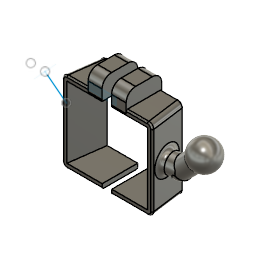
Titan_Grab_Bar_Monitor_Mount 2 v1.1 (Autodesk Fusion 360 design; units mm, degrees)
part number: 2026-08-07-00-05-41-022
Autodesk Fusion 360 part; units mm, degrees
sketch "Sketch1" plane through (0, 0, 0) normal (0, 0, 1) x (1, 0, 0)
  line L0 (19.05, -19.05) -> (-19.05, -19.05)
  line L1 (-19.05, -19.05) -> (-19.05, 19.05)
  line L2 (-19.05, 19.05) -> (19.05, 19.05)
  line L3 (19.05, 19.05) -> (19.05, -19.05)
  line L4 (19.05, -19.05) -> (-19.05, 19.05) construction
  line L5 (-19.05, -19.05) -> (19.05, 19.05) construction
  dimension "d8" = 38.1
  dimension "d9" = 38.1
  constraint horizontal L0
  constraint perpendicular L0 L1
  constraint parallel L0 L2
  constraint parallel L1 L3
  constraint coincident L4 origin
  constraint coincident L5 origin
  measures "d8" distance of L1.end L2.end
  measures "d9" distance of L0.end L1.end
ref_plane "WorkPlane1" through (0, 0, 19.05) normal (0, 0, 1) x (1, 0, 0)
sketch "Sketch2" plane through (0, 0, 19.05) normal (0, 0, 1) x (1, 0, 0)
  line L0 (16.51, 19.05) -> (-16.51, 19.05)
  line L1 (-16.51, 19.05) -> (-16.51, -19.05)
  line L2 (-16.51, -19.05) -> (16.51, -19.05)
  line L3 (16.51, -19.05) -> (16.51, 19.05)
  line L4 (16.51, 19.05) -> (-16.51, -19.05) construction
  line L5 (-16.51, 19.05) -> (16.51, -19.05) construction
  dimension "d12" = 33.02
  dimension "d13" = 38.1
  constraint horizontal L0
  constraint perpendicular L0 L1
  constraint parallel L0 L2
  constraint parallel L1 L3
  constraint coincident L4 origin
  constraint coincident L5 origin
  measures "d12" distance of L1.end L2.end
  measures "d13" distance of L0.end L1.end
loft "Loft1" add profiles "Sketch1", "Sketch2" section 1 section 2 makes body 1
shell "Shell3" thickness 2.54 outward yes removed faces 2 at (5.5033, -6.35, 19.05) at (-6.35, 6.35, 0) on bodies 1
fillet "Fillet1" radius 2.54 4 edges at (-20.3425, 21.59, 9.525) (20.3425, 21.59, 9.525) (20.3425, -21.59, 9.525) (-20.3425, -21.59, 9.525) on bodies 1
fillet "Fillet2" radius 0.762 24 edges at (19.0725, 0, 19.05) (18.3219, -20.8461, 19.05) (0, -21.59, 19.05) (-18.3219, -20.8461, 19.05) (-19.0725, 0, 19.05) (-18.3219, 20.8461, 19.05) (0, 21.59, 19.05) (18.3219, 20.8461, 19.05) (20.8619, 20.8461, 0) (21.6125, 0, 0) (20.8619, -20.8461, 0) (0, -21.59, 0) (-20.8619, -20.8461, 0) (-21.6125, 0, 0) (-20.8619, 20.8461, 0) (0, 21.59, 0) (20.8619, -20.8461, 0) (0, -21.59, 0) (-20.8619, -20.8461, 0) (-21.6125, 0, 0) (-20.8619, 20.8461, 0) (0, 21.59, 0) (20.8619, 20.8461, 0) (21.6125, 0, 0) on bodies 1
ref_plane "WorkPlane2" through (0, 0, 8.1748) normal (1, 0, 0) x (0, 0, -1)
sketch "Sketch3" plane through (0, 0, 0) normal (1, 0, 0) x (0, 0, -1)
  line L0 (-19.0413, 19.7767) -> (0.0528, 19.7767)
  line L1 (0.0528, 19.7767) -> (0.0528, 29.9367)
  line L2 (0.0528, 29.9367) -> (-19.0413, 29.9367)
  line L3 (-19.0413, 29.9367) -> (-19.0413, 19.7767)
  dimension "d22" = 10.16
  constraint horizontal L0
  constraint vertical L1
  constraint horizontal L2
  constraint vertical L3
  measures "d22" distance of L0.start L2.end
extrude "Extrude1" add sketch "Sketch3" along normal blind 7.62 and the other way blind 7.62 bodies 1
fillet "Fillet3" radius 5.08 2 edges at (0, 29.9367, 19.0413) (0, 29.9367, -0.0528) on bodies 1
ref_plane "WorkPlane3" through (-19.1607, 19.05, 18.3887) normal (-0.991228, 0, 0.132164) x (0, -1, 0)
sketch "Sketch4" plane through (-21.235, 0, 2.8313) normal (-0.991228, 0, 0.132164) x (0, -1, 0)
  circle A0 centre (0, 6.2571) radius 5.08
  dimension "d32" = 10.16
  measures "d32" diameter of A0
extrude "Extrude2" add sketch "Sketch4" along normal blind 7.62 bodies 1
ref_plane "WorkPlane4" through (-40.5498, 0, 11.7191) normal (-0.991228, 0, 0.132164) x (0, -1, 0)
sketch "Sketch5" plane through (0, 0, 19.0413) normal (0, 0, 1) x (1, 0, 0)
  line L0 (7.62, 24.8567) -> (-7.62, 24.8567)
  line L1 (-7.62, 24.8567) -> (-7.62, 20.9426)
  line L2 (-7.62, 20.9426) -> (7.62, 20.9426)
  line L3 (7.62, 20.9426) -> (7.62, 24.8567)
  point P0 (-38.1, 17.78)
sketch "Sketch6" plane through (-21.235, 0, 2.8313) normal (-0.991228, 0, 0.132164) x (0, -1, 0)
  line L0 (-10.16, 6.35, 17.78) -> (0, 6.35, 7.62)
  point P0 (0, 6.35)
ref_plane "WorkPlane5" through (-38.0198, 10.16, 11.4755) normal (0.700904, -0.707107, -0.093454) x (0.710215, 0.703985, 0)
sketch "Sketch7" plane through (-38.0198, 10.16, 11.4755) normal (0.700904, -0.707107, -0.093454) x (0.710215, 0.703985, 0)
  circle A0 centre (0, 0) radius 5.08
  dimension "d38" = 10.16
  constraint coincident A0.centre origin
  measures "d38" diameter of A0
extrude "Extrude3" add sketch "Sketch7" along normal blind 20.32 bodies 1
sketch "Sketch8" plane through (0, 0, 0) normal (1, 0, 0) x (0, 0, -1)
fillet "Fillet4" radius 5.08 1 edges at (-27.3223, -7.7996, 10.1623) on bodies 1
sphereprimitive "SpherePrimitive1" [suppressed]
sketch "Sketch10" plane through (-24.4649, 24.6814, 3.262) normal (-0.700904, 0.707107, 0.093454) x (0.132164, 0, 0.991228)
  circle A0 centre (6.35, -20.5364) radius 5.08
sphere "SpherePrimitive2" add diameter 15.24 placed x (0.710215, 0.703985, 0) y (0.06579, -0.066372, 0.995624) z (0.700904, -0.707107, -0.093454) at (-38.0198, 10.16, 11.4755) bodies 1
move_body "Move2" bodies 1 to x (-1, 0, 0) y (0, 1, 0) z (0, 0, -1) at (0.1605, 0, 18.9444)
fillet "Fillet5" radius 2.54 1 edges at (20.3257, 4.7362, 8.09) on bodies 1
split "Split1" by plane through (0, 0, 8.1748) normal (1, 0, 0) bodies 1 makes body 2 at (18.3638, -6.35, 12.5944)
move_body "Move3" bodies 2 to x (1, 0, 0) y (0, 1, 0) z (0, 0, 1) at (5.08, 0, 0)
move_body "Move1" [rolled back]
shell "Shell1" [rolled back] inner thickness 2.54
shell "Shell2" [suppressed]
equation "W1 = 1.5 in"
equation "D1 = 1.5 in"
equation "W2 = 1.3 in"
equation "D2 = 1.5 in"
equation "ClampWidth = 0.75 in"
equation "ClampFillet = 0.3"
equation "clampWall = 0.2 in"
equation "d8 = W1"
equation "d9 = D1"
equation "d10 = ClampWidth"
equation "d12 = W2"
equation "d13 = D2"
equation "d22 = bossHeight"
equation "bossHeight = 0.4 in"
equation "shaftDiameter = 0.4 in"
equation "d32 = shaftDiameter"
equation "d38 = shaftDiameter"
named bodies: "Rear Clamp Shell", "Front Clamp Shell"
